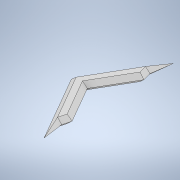
# Autodesk Inventor part: SpeedRank
Saved by Autodesk Inventor 2020 (Build 240168000, 168)
## iProperties
Created: 2020-01-12
Part Number: SpeedRank
Material: Generic
Document SubType Name: Modeling
Designer: atmat
Density: 1 g/cm^3
Appearance: Default
Author: atmat
Autodesk Inventor part; units mm, degrees
ref_plane "YZ Plane" through (0, 0, 0) normal (1, 0, 0) x (0, 1, 0)
ref_plane "XZ Plane" through (0, 0, 0) normal (0, 1, 0) x (-1, 0, 0)
ref_plane "XY Plane" through (0, 0, 0) normal (0, 0, 1) x (1, 0, 0)
sketch "Sketch1" plane through (0, 0, 0) normal (0, 1, 0) x (-1, 0, 0)
  line L0 (5.7735, 0) -> (-7.7265, 23.3827)
  line L1 (-7.7265, 23.3827) -> (-6.6962, 15.9904)
  line L2 (-6.6962, 15.9904) -> (-7.5, 12.9904)
  line L3 (-7.5, 12.9904) -> (0, 0)
  line L4 (0, 0) -> (-7.5, -12.9904)
  line L5 (-7.5, -12.9904) -> (-6.6962, -15.9904)
  line L6 (-6.6962, -15.9904) -> (-7.7265, -23.3827)
  line L7 (-7.7265, -23.3827) -> (5.7735, 0)
  line L8 (14.7308, 0) -> (-3.2807, 0) construction
  dimension "d0" = 0
  dimension "d1" = 0
  dimension "d2" = 0
  dimension "d3" = 60
  dimension "d4" = 60
  dimension "d5" = 5
  dimension "d6" = 135
  dimension "d7" = 135
  dimension "d8" = 15
  dimension "d9" = 15
  dimension "d10" = 3
  dimension "d11" = 3
  dimension "d12" = 27
  dimension "d13" = 27
  constraints: 18 end point, 2 parallel, 1 horizontal
  measures "d0" vertical distance of point (0, 0) L0.start
  measures "d1" distance of point (0, 0) L3.end
  measures "d2" distance of point (0, 0) L3.end
  measures "d3" angle of L0 L8
  measures "d4" angle of L7 L8
  measures "d5" distance between parallel lines of L3 L0
  measures "d6" angle of L4 L5
  measures "d7" angle of L2 L3
  measures "d8" distance of L2.end L3.end
  measures "d9" distance of L3.end L4.end
  measures "d10" vertical distance of L1.end L2.end
  measures "d11" vertical distance of L4.end L5.end
  measures "d12" distance of L0.start L0.end
  measures "d13" distance of L6.end L0.start
extrude "Extrusion1" add sketch "Sketch1" along normal blind 3
chamfer "Chamfer1" distance 1.5 angle 45 6 edges at (3.75, 3, 6.4952) (3.75, 3, -6.4952) (7.0981, 3, -14.4904) (7.0981, 3, 14.4904) (7.2113, 3, 19.6865) (7.2113, 3, -19.6865)
chamfer "Chamfer2" distance 1.5 angle 45 2 edges at (-0.0217, 3, 9.9623) (-0.0217, 3, -9.9623)
chamfer "Chamfer3" distance 1.5 angle 45 6 edges at (3.75, 0, -6.4952) (7.0981, 0, -14.4904) (7.2113, 0, -19.6865) (3.75, 0, 6.4952) (7.2113, 0, 19.6865) (7.0981, 0, 14.4904)
chamfer "Chamfer4" distance 1.5 angle 45 2 edges at (-0.0214, 0, -9.9629) (-0.0214, 0, 9.9629)
body "Solid1"
